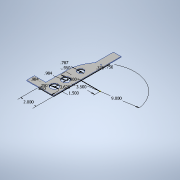
# Autodesk Inventor part: buttonpanel4.5
Saved by Autodesk Inventor 2021 (Build 250183000, 183)
## iProperties
Created: 2020-11-08
Part Number: buttonpanel4.5
Material: Aluminum 6061
Document SubType Name: Modeling
Designer: mackeycj
Density: 2.7 g/cm^3
Appearance: Aluminum - Flat
Mass: 54.1801 g
Surface Area: 195.326 cm^2
Volume: 20.0667 cm^3
Author: mackeycj
Autodesk Inventor part; units mm, degrees
ref_plane "YZ Plane" through (0, 0, 0) normal (1, 0, 0) x (0, 1, 0)
ref_plane "XZ Plane" through (0, 0, 0) normal (0, 1, 0) x (-1, 0, 0)
ref_plane "XY Plane" through (0, 0, 0) normal (0, 0, 1) x (1, 0, 0)
sketch "Sketch1" plane through (0, 0, 0) normal (0, 1, 0) x (-1, 0, 0)
  arc A0 (63.5, -95.0381) -> (114.3, 0) centre (0, 0) ccw
  line L0 (114.3, 0) -> (114.3, 91.948)
  line L1 (114.3, 91.948) -> (63.5, 91.948)
  line L2 (63.5, 91.948) -> (63.5, -95.0381)
  line L3 (0, 0) -> (88.9, 0)
  line L4 (88.9, 0) -> (88.9, -24.13)
  circle A1 centre (88.9, -24.13) radius 10
  line L5 (88.9, 0) -> (88.9, 25.4)
  circle A2 centre (88.9, 25.4) radius 12.4968
  line L6 (88.9, 25.4) -> (88.9, 63.5)
  circle A3 centre (88.9, 63.5) radius 12.4968
  line L7 (114.3, 91.948) -> (114.3, 85.598)
  line L8 (114.3, 85.598) -> (107.95, 85.598)
  line L9 (63.5, -95.0381) -> (63.5, -75.9881)
  line L10 (63.5, -75.9881) -> (73.025, -75.9881)
  dimension "d0" = 228.6
  dimension "d1" = 91.948
  dimension "d2" = 50.8
  dimension "d3" = 88.9
  dimension "d4" = 24.13
  dimension "d5" = 20
  dimension "d6" = 25.4
  dimension "d7" = 24.9936
  dimension "d8" = 38.1
  dimension "d9" = 24.9936
  dimension "d12" = 6.35
  dimension "d13" = 6.35
  dimension "d14" = 19.05
  dimension "d15" = 9.525
  constraints: 22 end point, 5 perpendicular, 4 centre point, 4 coincident, 3 vertical, 2 point on circle, 2 point on line, 1 horizontal, 1 tangent
  measures "d0" diameter of A0
  measures "d1" distance of L0.start L0.end
  measures "d2" distance of L0.end L1.end
  measures "d3" distance of L3.start L3.end
  measures "d4" distance of L3.end L4.end
  measures "d5" diameter of A1
  measures "d6" distance of L3.end L5.end
  measures "d7" diameter of A2
  measures "d8" distance of L6.start L6.end
  measures "d9" diameter of A3
  measures "d12" distance of L0.end L7.end
  measures "d13" distance of L7.end L8.end
  measures "d14" distance of L2.end L9.end
  measures "d15" distance of L9.end L10.end
extrude "Extrusion1" add sketch "Sketch1" along normal blind 2.286
hole "Hole1" at (-107.95, 0, 85.598) at (-73.025, 0, -75.9881) direction (0, 1, 0) diameter 3.2766 end through all clearance for "Flat Head Machine Screw (82)" size "#4" standard "Ansi Unified Screw Threads"
sketch "Sketch2" plane through (0, 0, 0) normal (0, 1, 0) x (-1, 0, 0)
  line L0 (0, 0) -> (63.5, 0)
  line L1 (63.5, 91.948) -> (63.5, -95.0381) projected
  line L2 (114.3, 91.948) -> (63.5, 91.948) projected
  line L3 (63.5, 91.948) -> (114.3, 91.948)
  line L4 (114.3, 91.948) -> (152.4, 91.948)
  line L5 (152.4, 91.948) -> (152.4, 66.548)
  line L6 (152.4, 66.548) -> (114.3, 66.548)
  line L7 (114.3, 66.548) -> (114.3, 91.948)
  arc A0 (63.5, -95.0381) -> (114.3, 0) centre (0, 0) ccw projected
  line L8 (63.5, -95.0381) -> (88.9, -95.0381)
  line L9 (88.9, -95.0381) -> (88.9, -71.842)
  line L10 (88.9, -95.0381) -> (63.5, -95.0381)
  line L11 (63.5, -95.0381) -> (63.5, -133.1381)
  line L12 (63.5, -133.1381) -> (88.9, -133.1381)
  line L13 (88.9, -133.1381) -> (88.9, -95.0381)
  line L14 (76.2, -95.0381) -> (76.2, -126.7881)
  line L15 (114.3, 0) -> (114.3, 91.948) projected
  line L16 (114.3, 79.248) -> (114.3, 47.498)
  line L17 (114.3, 79.248) -> (146.05, 79.248)
  line L18 (114.3, 79.248) -> (146.05, 79.248) construction
  dimension "d23" = 38.1
  dimension "d24" = 25.4
  dimension "d25" = 25.4
  dimension "d26" = 25.4
  dimension "d27" = 38.1
  dimension "d28" = 31.75
  dimension "d29" = 31.75
  dimension "d30" = 31.75
  constraints: 32 end point, 5 equal length, 5 horizontal, 4 perpendicular, 3 point on line, 1 collinear, 1 midpoint, 1 point on circle, 1 vertical
  measures "d23" distance of L5.end L6.end
  measures "d24" distance of L4.end L5.end
  measures "d25" distance of L1.end L8.end
  measures "d26" distance of L12.end L11.end
  measures "d27" distance of L11.end L10.end
  measures "d28" distance of L14.start L14.end
  measures "d29" distance of L16.start L16.end
  measures "d30" distance of L16.start L17.end
extrude "Extrusion2" add sketch "Sketch2" along normal blind 2.286 contours L4 L5 L6 L7 | A0 L9 L8 | L8 L13 L12 L11
body "Solid1"
